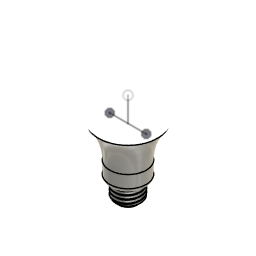
day9-light_bulb (Autodesk Fusion 360 design; units mm, degrees)
part number: 2025-06-22-19-40-50-722
part number: 2025-06-22-19-44-19-735
Autodesk Fusion 360 part; units mm, degrees
cylinder "CylinderPrimitive1" add diameter 30 height 40 placed x (1, 0, 0) y (0, 1, 0) z (0, 0, 1) at (0, 0, 0) makes body 1 in component "lightBulb1"
sketch "Sketch2" plane through (0, 0, 0) normal (0, 1, 0) x (1, 0, 0) in component "lightBulb1"
  line L0 (-15, -40) -> (15, -40)
  line L1 (0, -40) -> (0, -60)
  point P0 (-15, -40)
  point P1 (15, -40)
  constraint coincident P0 L0.start
  constraint coincident P1 L0.end
  constraint midpoint L0 L1.start
  constraint perpendicular L0 L1
sphere "SpherePrimitive1" add diameter 61 placed x (1, 0, 0) y (0, 0, -1) z (0, 1, 0) at (0, 0, 60) bodies 1 in component "lightBulb1"
fillet "Fillet1" radius 45 1 edges at (-13.9849, 5.4242, 33.4435) on bodies 1 in component "lightBulb1"
fillet "Fillet1" radius 4 1 edges at (-13.9849, 5.4242, 0) on bodies 1 in component "lightBulb1"
cylinder "CylinderPrimitive2" add diameter 22 height -15 placed x (1, 0, 0) y (0, 1, 0) z (0, 0, 1) at (0, 0, 0) separate body makes body 2 in component "lightBulb1"
thread "Thread1" "ISO Metric profile 22.0 M22x3 M22x3 6g" major diameter 21.7645 minor diameter 18.3374 pitch 3 angle 60 modelled right hand crest width 0.4298 on face at (10.9453, -1.0952, -10) from (0, 0, 0) to (0, 0, -12) crest through (0, 10.8823, 0.75) on bodies 2 in component "lightBulb1"
chamfer "Chamfer1" distance 4 angle 45 1 edges at (-3.9352, -10.1458, -15) measured on face at (2.3404, -0.3528, -15) on bodies 2 in component "lightBulb1"
fillet "Fillet2" radius 2 1 edges at (2.4887, -6.4165, -15) on bodies 2 in component "lightBulb1"
sketch "Sketch5" plane through (0, 0, 0) normal (1, 0, 0) x (0, 1, 0) in component "lightBulb1"
cylinder "CylinderPrimitive3" add diameter 10.212 height 2 placed x (0, 1, 0) y (1, 0, 0) z (0, 0, -1) at (0, 0, -15) separate body makes body 3 in component "lightBulb1"
chamfer "Chamfer2" distance 2 angle 45 1 edges at (-1.8464, -4.7605, -17) measured on face at (0.7857, -1.2198, -17) on bodies 3 in component "lightBulb1"
component "lightBulb1" placed x (1, 0, 0) y (0, 1, 0) z (0, 0, 1) at (0, 0, 0)
